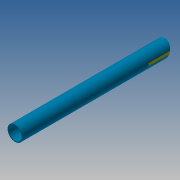
# Autodesk Inventor part: 2p5vss
Saved by Autodesk Inventor 2014 SP1 (Build 180222100, 222)
## iProperties
Company: HERA Project
Created: 2013-06-11
Part Number: 2p5vss
Material: PVC-Piping
Document SubType Name: Modeling
Designer: David DeBoer
Density: 1.4 g/cm^3
Description: support vertical spar
Mass: 468.384 g
Surface Area: 1724.47 cm^2
Volume: 334.56 cm^3
Appearance: Smooth - White
Author: David DeBoer
Title: Hub-supporthold
Autodesk Inventor part; units mm, degrees
sketch "Sketch1" plane through (0, 0, 0) normal (0, 0, 1) x (1, 0, 0)
  circle A0 centre (0, 0) radius 31.5
  circle A1 centre (0, 0) radius 27.5
  dimension "d0" = 63
  dimension "d2" = 4
  constraints: 2 centre point, 1 coincident
  measures "d0" diameter of A0
  measures "d2" radial gap between concentric circles of A1 A0
extrude "tube" add sketch "Sketch1" along normal blind 627
sketch "Sketch15" plane through (0, 0, 627) normal (0, 0, 1) x (1, 0, 0)
  circle A0 centre (0, 0) radius 27.5 projected
  circle A1 centre (0, 0) radius 31.5 projected
  point P0 (31.5, 0)
  constraints: 1 horizontal alignment, 1 other
ref_plane "Work Plane6" through (31.5, 0, 627) normal (1, 0, 0) x (0, 1, 0)
ref_plane "Work Plane7" through (31, 0, 0) normal (1, 0, 0) x (0, 1, 0)
sketch "Sketch19" plane through (31, 0, 0) normal (1, 0, 0) x (0, 1, 0)
  line L0 (-10, 0) -> (10, 0)
  line L1 (10, 0) -> (10, 100)
  line L2 (10, 100) -> (-10, 100)
  line L3 (-10, 100) -> (-10, 0)
  point P0 (0, 0)
  point P1 (0, 0)
  dimension "d67" = 20
  dimension "d68" = 100
  constraints: 8 end point, 2 parallel, 1 coincident, 1 horizontal, 1 midpoint, 1 perpendicular
  measures "d67" distance of L2.end L1.end
  measures "d68" distance of L1.end L0.end
extrude "flatFaceYellow" cut sketch "Sketch19" along normal blind 25.4
sketch "Sketch21" plane through (0, 0, 0) normal (0, 0, -1) x (-1, 0, 0)
  line L0 (-31, 5.5902) -> (-31, -5.5902) projected
  arc A0 (-31, -5.5902) -> (-31, 5.5902) centre (0, 0) ccw projected
  circle A1 centre (0, 0) radius 27.5 projected
  line L1 (0.7293, 31.4916) -> (30.8537, 31.4916) construction
  constraints: 2 end point, 1 perpendicular, 1 point on circle
ref_plane "Work Plane8" through (-0.7293, 31.4916, 0) normal (0, -0.3387, -0.9409) x (-1, 0, 0)
sketch "Sketch22" plane through (-0.7293, 31.4916, 0) normal (0, -0.3387, -0.9409) x (-1, 0, 0)
  line L0 (-34.8075, -84.5558) -> (31.7452, -84.5558)
  line L1 (31.7452, -84.5558) -> (31.7452, 8.8585)
  line L2 (31.7452, 8.8585) -> (-34.8075, 8.8585)
  line L3 (-34.8075, 8.8585) -> (-34.8075, -84.5558)
  point P0 (-0.7293, -29.6298)
  constraints: 8 end point, 2 parallel, 1 horizontal, 1 perpendicular
extrude "angledEnd" cut sketch "Sketch22" along normal blind 25.4
sketch "Sketch23" plane through (31, 0, 0) normal (1, 0, 0) x (0, 0, -1)
  line L0 (-13.3502, -5.5902) -> (-100, -5.5902) projected
  circle A0 centre (-80, 0) radius 3.2074
  circle A1 centre (-40, 0) radius 3.2074
  point P0 (0, 0)
  dimension "d89" = 80
  dimension "d92" = 40
  constraints: 2 centre point, 1 horizontal, 2 other
  measures "d89" distance of A0.centre point (0, 0)
  measures "d92" distance of A0.centre A1.centre
hole "Hole3" at (31, 0, 80) at (31, 0, 40) direction (-1, 0, 0) diameter 2 end through all
body "Solid1"
